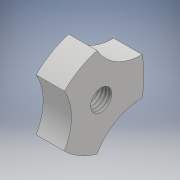
# Autodesk Inventor part: 零件4
Saved by Autodesk Inventor 2018 (Build 220112000, 112)
## iProperties
Created: 2023-04-30
Part Number: 零件4
Material: 常规
Document SubType Name: Sheet Metal
Designer: 47376
Density: 1 g/cm^3
Sheet Metal Rule: 默认_mm
Appearance: 默认
Author: 47376
Autodesk Inventor part; units mm, degrees
ref_plane "YZ Plane" through (0, 0, 0) normal (1, 0, 0) x (0, 1, 0)
ref_plane "XZ Plane" through (0, 0, 0) normal (0, 1, 0) x (-1, 0, 0)
ref_plane "XY Plane" through (0, 0, 0) normal (0, 0, 1) x (1, 0, 0)
sketch "草图1" plane through (0, 0, 0) normal (1, 0, 0) x (0, 1, 0)
  point P0 (0, 0)
sketch "草图2" plane through (0, 0, 0) normal (1, 0, 0) x (0, 1, 0)
  circle A0 centre (0, 0) radius 2.25
  arc A1 (-7.7942, -5.5) -> (-7.7942, 5.5) centre (-17.1276, 0) ccw
  arc A2 (-0.866, 9.5) -> (8.6603, 4) centre (8.5638, 14.8329) ccw
  arc A3 (8.6603, -4) -> (-0.866, -9.5) centre (8.5638, -14.8329) ccw
  arc A4 (8.6603, -4) -> (8.6603, 4) centre (-10.9632, 0) ccw
  arc A5 (-0.866, 9.5) -> (-7.7942, 5.5) centre (3.5449, -6.1399) ccw
  arc A6 (-7.7942, -5.5) -> (-0.866, -9.5) centre (3.5449, 6.1399) ccw
  dimension "d0" = 4.5
  constraints: 12 point on circle, 7 centre point, 1 coincident, 1 other
  measures "d0" diameter of A0
extrude "拉伸1" add sketch "草图2" along normal blind 6
thread "螺纹1" size "M4.5x0.75" class "6H" standard "ANSI Metric M Profile" full length
equation "\"折弯半径\" = 厚度"
equation "\"折弯释压宽度\" = 厚度"
equation "\"折弯释压深度\" = 0.5 * 厚度"
equation "\"拐角释压尺寸\" = 4 * 厚度"
equation "\"最小余量\" = 2 * 厚度"
equation "\"过渡半径\" = 折弯半径"
equation "\"Jacobi半径尺寸\" = 折弯半径"
equation "\"间隙大小\" = 厚度"
equation "\"厚度\" = 0.5"
